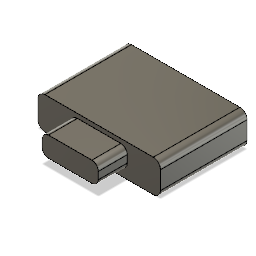
LED retaining Peg v1 (Autodesk Fusion 360 design; units mm, degrees)
Autodesk Fusion 360 part; units mm, degrees
sketch "Sketch1" plane through (0, 0, 0) normal (0, 0, 1) x (1, 0, 0)
  line L0 (8.5, 2.25) -> (-8.5, 2.25)
  line L1 (-8.5, 2.25) -> (-8.5, -2.25)
  line L2 (-8.5, -2.25) -> (8.5, -2.25)
  line L3 (8.5, -2.25) -> (8.5, 2.25)
  line L4 (8.5, 2.25) -> (-8.5, -2.25) construction
  line L5 (-8.5, 2.25) -> (8.5, -2.25) construction
  dimension "d1" = 17
  dimension "d2" = 4.5
  constraint horizontal L0
  constraint perpendicular L0 L1
  constraint parallel L0 L2
  constraint parallel L1 L3
  constraint coincident L4 origin
  constraint coincident L5 origin
  measures "d1" distance of L1.end L2.end
  measures "d2" distance of L0.end L1.end
extrude "Extrude1" add sketch "Sketch1" along normal blind 12
sketch "Sketch2" plane through (0, 0, 12) normal (0, 0, 1) x (1, 0, 0)
  line L0 (8.5, -2.25) -> (8.5, 2.25)
  line L1 (8.5, 2.25) -> (-8.5, 2.25)
  line L2 (-8.5, 2.25) -> (-8.5, -2.25)
  line L3 (-8.5, -2.25) -> (8.5, -2.25)
  line L4 (3.9, 1.65) -> (-3.9, 1.65)
  line L5 (-3.9, 1.65) -> (-3.9, -1.15)
  line L6 (-3.9, -1.15) -> (3.9, -1.15)
  line L7 (3.9, -1.15) -> (3.9, 1.65)
  line L8 (3.9, 1.65) -> (-3.9, -1.15) construction
  line L9 (-3.9, 1.65) -> (3.9, -1.15) construction
  point P0 (0, 0.25)
  dimension "d5" = 7.8
  dimension "d6" = 2.8
  dimension "d7" = 0.6
  constraint horizontal L4
  constraint perpendicular L4 L5
  constraint parallel L4 L6
  constraint parallel L5 L7
  constraint coincident L8 P0
  constraint coincident L9 P0
  constraint vertical origin P0
  measures "d5" distance of L4.start L4.end
  measures "d6" distance of L4.start L6.end
  measures "d7" distance of L1 L4
extrude "Extrude2" add sketch "Sketch2" along normal blind 4 contours L4 L5 L6 L7
fillet "Fillet1" radius 1 4 edges at (-8.5, 2.25, 6) (-8.5, -2.25, 6) (8.5, -2.25, 6) (8.5, 2.25, 6)
fillet "Fillet2" radius 0.9 4 edges at (3.9, 1.65, 14) (-3.9, 1.65, 14) (3.9, -1.15, 14) (-3.9, -1.15, 14)
